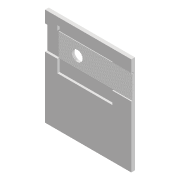
# Autodesk Inventor part: 00_cellSTORM_chip_01_old
Saved by Autodesk Inventor 2022 (Build 260153000, 153)
## iProperties
Created: 2020-05-10
Part Number: 00_cellSTORM_chip_01_old
Material: Generic
Document SubType Name: Modeling
Designer: diederichbenedict
Density: 1 g/cm^3
Appearance: Default
Author: diederichbenedict
Autodesk Inventor part; units mm, degrees
ref_plane "YZ Plane" through (0, 0, 0) normal (1, 0, 0) x (0, 1, 0)
ref_plane "XZ Plane" through (0, 0, 0) normal (0, 1, 0) x (-1, 0, 0)
ref_plane "XY Plane" through (0, 0, 0) normal (0, 0, 1) x (1, 0, 0)
sketch "Sketch1" plane through (0, 0, 0) normal (0, 0, 1) x (1, 0, 0)
  line L0 (0, 0) -> (23.76, 0)
  line L1 (23.76, 0) -> (23.76, 27)
  line L2 (23.76, 27) -> (0, 27)
  line L3 (0, 27) -> (0, 0)
  dimension "d0" = 23.76
  dimension "d1" = 27
  constraints: 8 end point, 2 parallel, 1 horizontal, 1 perpendicular
  measures "d0" distance of L2.end L1.end
  measures "d1" distance of L1.end L0.end
extrude "Extrusion1" add sketch "Sketch1" along normal blind 1
sketch "Sketch2" plane through (0, 0, 1) normal (0, 0, 1) x (1, 0, 0)
  line L0 (0, 0) -> (23.76, 0) projected
  line L1 (23.76, 0) -> (23.76, 27) projected
  line L2 (23.76, 27) -> (0, 27) projected
  line L3 (0, 27) -> (0, 0) projected
  line L4 (23.76, 0) -> (23.76, 27) projected
  line L5 (0, 23.7) -> (23.76, 23.7)
  line L6 (23.76, 23.7) -> (23.76, 16.95)
  line L7 (23.76, 16.95) -> (0, 16.95)
  line L8 (0, 16.95) -> (0, 23.7)
  line L9 (3.4, 24.9714) -> (18.51, 24.9714)
  line L10 (18.51, 24.9714) -> (18.51, 13.5)
  line L11 (18.51, 13.5) -> (3.4, 13.5)
  line L12 (3.4, 13.5) -> (3.4, 24.9714)
  dimension "d4" = 6.75
  dimension "d5" = 3.3
  dimension "d9" = 3.4
  dimension "d10" = 5.25
  constraints: 16 end point, 4 parallel, 2 horizontal, 2 perpendicular, 2 point on line
  measures "d4" distance of L5.end L6.end
  measures "d5" distance between parallel lines of L5 L2
  measures "d9" distance between parallel lines of L12 L3
  measures "d10" distance between parallel lines of L1 L10
extrude "Extrusion2" cut sketch "Sketch2" against normal blind 0.6 contours L3 L5 L12 L7 | L7 L10 L5 L1 | L12 L5 L10 L7 | L7 L10 L11 L12 | L12 L9 L10 L5
sketch "Sketch3" plane through (23.76, 0, 0) normal (1, 0, 0) x (0, 0, -1)
  line L0 (-0.4, 16.95) -> (-1, 16.95) projected
  line L1 (-1, 0) -> (-1, 16.95) projected
  line L2 (0, 0) -> (-1, 0) projected
  line L3 (0, 0) -> (0, 27) projected
  line L4 (0, 27) -> (-1, 27) projected
  line L5 (-1, 23.7) -> (-1, 27) projected
  line L6 (-1, 23.7) -> (-0.4, 23.7) projected
  line L7 (-0.4, 23.7) -> (-0.4, 16.95) projected
  circle A0 centre (-0.5521, 23.2257) radius 0.1521
  line L8 (-0.4, 23.7) -> (-0.4, 16.95) projected
  point P0 (0, 0)
  constraints: 1 centre point, 1 tangent
extrude "Extrusion3" add sketch "Sketch3" against normal up to surface (20.36 mm away) contours A0
pattern_linear "Rectangular Pattern1" count 24 spacing 0.27 along (0, -1, 0) of "Extrusion3"
sketch "Sketch4" plane through (0, 0, 1) normal (0, 0, 1) x (1, 0, 0)
  line L0 (3.4, 16.95) -> (0, 16.95) projected
  line L1 (3.4, 13.5) -> (3.4, 16.95) projected
  line L2 (18.51, 13.5) -> (3.4, 13.5) projected
  line L3 (18.51, 16.95) -> (18.51, 13.5) projected
  line L4 (23.76, 16.95) -> (18.51, 16.95) projected
  line L5 (23.76, 17.0157) -> (23.76, 16.95) projected
  line L6 (23.76, 17.0157) -> (3.4, 17.0157) projected
  line L7 (23.76, 17.2857) -> (23.76, 17.0157) projected
  line L8 (23.76, 17.2857) -> (3.4, 17.2857) projected
  line L9 (23.76, 17.5557) -> (23.76, 17.2857) projected
  line L10 (23.76, 17.5557) -> (3.4, 17.5557) projected
  line L11 (23.76, 17.8257) -> (23.76, 17.5557) projected
  line L12 (23.76, 17.8257) -> (3.4, 17.8257) projected
  line L13 (23.76, 18.0957) -> (23.76, 17.8257) projected
  line L14 (23.76, 18.0957) -> (3.4, 18.0957) projected
  line L15 (23.76, 18.3657) -> (23.76, 18.0957) projected
  line L16 (23.76, 18.3657) -> (3.4, 18.3657) projected
  line L17 (23.76, 18.6357) -> (23.76, 18.3657) projected
  line L18 (23.76, 18.6357) -> (3.4, 18.6357) projected
  line L19 (23.76, 18.9057) -> (23.76, 18.6357) projected
  line L20 (23.76, 18.9057) -> (3.4, 18.9057) projected
  line L21 (23.76, 19.1757) -> (23.76, 18.9057) projected
  line L22 (23.76, 19.1757) -> (3.4, 19.1757) projected
  line L23 (23.76, 19.4457) -> (23.76, 19.1757) projected
  line L24 (23.76, 19.4457) -> (3.4, 19.4457) projected
  line L25 (23.76, 19.7157) -> (23.76, 19.4457) projected
  line L26 (23.76, 19.7157) -> (3.4, 19.7157) projected
  line L27 (23.76, 19.9857) -> (23.76, 19.7157) projected
  line L28 (23.76, 19.9857) -> (3.4, 19.9857) projected
  line L29 (23.76, 20.2557) -> (23.76, 19.9857) projected
  line L30 (23.76, 20.2557) -> (3.4, 20.2557) projected
  line L31 (23.76, 20.5257) -> (23.76, 20.2557) projected
  line L32 (23.76, 20.5257) -> (3.4, 20.5257) projected
  line L33 (23.76, 20.7957) -> (23.76, 20.5257) projected
  line L34 (23.76, 20.7957) -> (3.4, 20.7957) projected
  line L35 (23.76, 21.0657) -> (23.76, 20.7957) projected
  line L36 (23.76, 21.0657) -> (3.4, 21.0657) projected
  line L37 (23.76, 21.3357) -> (23.76, 21.0657) projected
  line L38 (23.76, 21.3357) -> (3.4, 21.3357) projected
  line L39 (23.76, 21.6057) -> (23.76, 21.3357) projected
  line L40 (23.76, 21.6057) -> (3.4, 21.6057) projected
  line L41 (23.76, 21.8757) -> (23.76, 21.6057) projected
  line L42 (23.76, 21.8757) -> (3.4, 21.8757) projected
  line L43 (23.76, 22.1457) -> (23.76, 21.8757) projected
  line L44 (23.76, 22.1457) -> (3.4, 22.1457) projected
  line L45 (23.76, 22.4157) -> (23.76, 22.1457) projected
  line L46 (23.76, 22.4157) -> (3.4, 22.4157) projected
  line L47 (23.76, 22.6857) -> (23.76, 22.4157) projected
  line L48 (23.76, 22.6857) -> (3.4, 22.6857) projected
  line L49 (23.76, 22.9557) -> (23.76, 22.6857) projected
  line L50 (23.76, 22.9557) -> (3.4, 22.9557) projected
  line L51 (23.76, 23.2257) -> (23.76, 22.9557) projected
  line L52 (23.76, 23.2257) -> (3.4, 23.2257) projected
  line L53 (23.76, 23.7) -> (23.76, 23.2257) projected
  line L54 (18.51, 23.7) -> (23.76, 23.7) projected
  line L55 (18.51, 24.9714) -> (18.51, 23.7) projected
  line L56 (3.4, 24.9714) -> (18.51, 24.9714) projected
  line L57 (3.4, 23.7) -> (3.4, 24.9714) projected
  line L58 (0, 23.7) -> (3.4, 23.7) projected
  line L59 (0, 16.95) -> (0, 23.7) projected
  circle A0 centre (8.5565, 20.0809) radius 1.4452
  point P0 (0, 0)
  constraints: 1 centre point, 1 tangent
extrude "Extrusion4" cut sketch "Sketch4" against normal blind 10 contours A0 L20 | A0 L22 L20 | A0 L24 L22 | A0 L26 L24 | A0 L36 L38 | L38 A0 | A0 L28 L26 | A0 L34 L36 | A0 L30 L28 | A0 L32 L34 | A0 L32 L30
body "Solid1"
